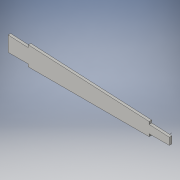
# Autodesk Inventor part: side board
Saved by Autodesk Inventor 2016 SP2 (Build 200236200, 236)
## iProperties
Created: 2017-09-04
Part Number: side board
Material: Generic
Document SubType Name: Modeling
Designer: Kartikye
Density: 1 g/cm^3
Appearance: Default
Author: Kartikye
Autodesk Inventor part; units mm, degrees
ref_plane "YZ Plane" through (0, 0, 0) normal (1, 0, 0) x (0, 1, 0)
ref_plane "XZ Plane" through (0, 0, 0) normal (0, 1, 0) x (-1, 0, 0)
ref_plane "XY Plane" through (0, 0, 0) normal (0, 0, 1) x (1, 0, 0)
sketch "Sketch1" plane through (0, 0, 0) normal (0, 0, 1) x (1, 0, 0)
  line L0 (-101.6, -12.7) -> (101.6, -12.7)
  line L1 (101.6, -12.7) -> (101.6, 12.7)
  line L2 (101.6, 12.7) -> (-101.6, 12.7)
  line L3 (-101.6, 12.7) -> (-101.6, -12.7)
  line L4 (-101.6, -12.7) -> (101.6, 12.7) construction
  line L5 (101.6, -12.7) -> (-101.6, 12.7) construction
  point P0 (0, 0)
  dimension "d0" = 203.2
  dimension "d1" = 25.4
  constraints: 12 end point, 2 midpoint, 2 parallel, 1 horizontal, 1 perpendicular
  measures "d0" distance of L2.end L1.end
  measures "d1" distance of L1.end L0.end
extrude "Extrusion1" add sketch "Sketch1" along normal blind 3.175
sketch "Sketch2" plane through (0, 0, 3.175) normal (0, 0, 1) x (1, 0, 0)
  line L0 (-101.6, -12.7) -> (101.6, -12.7) projected
  line L1 (-101.6, 12.6386) -> (101.5996, 2.54)
  line L2 (-101.6, 12.6386) -> (-115.0985, 49.6806)
  line L3 (-115.0985, 49.6806) -> (129.2537, 40.5846)
  line L4 (129.2537, 40.5846) -> (101.5996, 2.54)
  point P0 (0, 0)
  dimension "d4" = 15.24
  constraints: 8 end point
  measures "d4" distance from line of L0 L1.end
extrude "Extrusion2" cut sketch "Sketch2" against normal blind 3.175
sketch "Sketch3" plane through (0, 0, 3.175) normal (0, 0, 1) x (1, 0, 0)
  line L0 (-76.2, 11.3763) -> (-78.9338, 11.5121)
  line L1 (-76.2, 11.3763) -> (-76.3576, 8.2052)
  line L2 (76.1996, 3.8023) -> (76.042, 0.6312)
  line L3 (-76.3576, 8.2052) -> (-113.4193, 10.0471)
  line L4 (-101.6, 12.6386) -> (-113.4193, 10.0471)
  line L5 (76.042, 0.6312) -> (108.1145, -0.9627)
  line L6 (101.5996, 2.54) -> (108.1145, -0.9627)
  line L7 (-76.2, 11.3763) -> (-101.6, 12.6386)
  line L8 (76.1996, 3.8023) -> (101.5996, 2.54)
  point P0 (0, 0)
  point P1 (-81.4529, 11.6373)
  point P2 (-101.6, -12.7664)
  dimension "d7" = 25.4
  dimension "d8" = 3.175
  dimension "d10" = 25.4
  dimension "d11" = 3.175
  dimension "d13" = 90
  dimension "d14" = 90
  constraints: 18 end point, 2 coincident
  measures "d7" horizontal distance of L0.start L4.start
  measures "d8" distance of L1.end L0.start
  measures "d10" horizontal distance of L6.start L2.start
  measures "d11" distance of L2.start L2.end
  measures "d13" angle of L1 L3
  measures "d14" angle of L5 L2
extrude "Extrusion3" cut sketch "Sketch3" against normal blind 3.175
sketch "Sketch4" plane through (0, 0, 3.175) normal (0, 0, 1) x (1, 0, 0)
  line L0 (-101.6, -12.7) -> (-101.6, -9.525)
  line L1 (-101.6, -9.525) -> (-76.2, -9.525)
  line L2 (-76.2, -9.525) -> (-76.2, -12.7)
  line L3 (-76.2, -12.7) -> (-101.6, -12.7)
  line L4 (101.6, -12.7) -> (76.2, -12.7)
  line L5 (76.2, -12.7) -> (76.2, -9.525)
  line L6 (76.2, -9.525) -> (101.6, -9.525)
  line L7 (101.6, -12.7) -> (101.6, -0.6389) projected
  line L8 (101.6, -9.525) -> (101.6, -12.7)
  point P0 (0, 0)
  constraints: 16 end point, 3 perpendicular, 3 point on line, 1 collinear
extrude "Extrusion4" cut sketch "Sketch4" against normal blind 3.175
body "Solid1"
